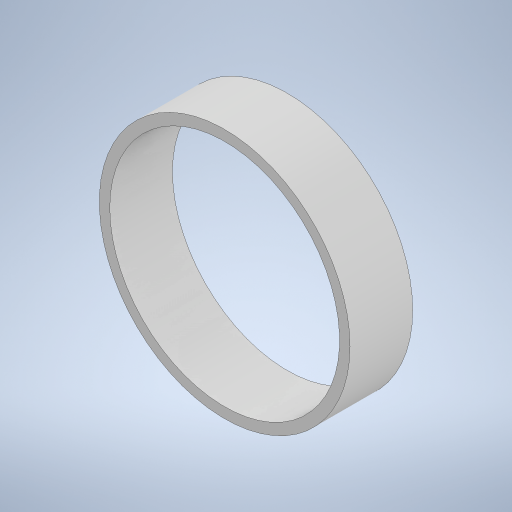
# Autodesk Inventor part: Ring Base
Saved by Autodesk Inventor 2024 (Build 280153000, 153)
## iProperties
Created: 2024-10-03
Part Number: Ring Base
Material: Generic
Document SubType Name: Modeling
Designer: Malik
Density: 1 g/cm^3
Appearance: Default
Author: Malik
Autodesk Inventor part; units mm, degrees
ref_plane "YZ Plane" through (0, 0, 0) normal (1, 0, 0) x (0, 1, 0)
ref_plane "XZ Plane" through (0, 0, 0) normal (0, 1, 0) x (-1, 0, 0)
ref_plane "XY Plane" through (0, 0, 0) normal (0, 0, 1) x (1, 0, 0)
sketch "Sketch1" plane through (0, 0, 0) normal (0, 0, 1) x (1, 0, 0)
  circle A0 centre (0, 0) radius 152.4
  dimension "d0" = 304.8
  constraints: 1 centre point, 1 coincident
  measures "d0" diameter of A0
extrude "Extrusion1" add sketch "Sketch1" along normal blind 76.2
shell "Shell1" thickness 12.7 removed faces 2 at (29.7836, -25.8225, 0) at (29.7836, -25.8225, 76.2)
body "Solid1"
